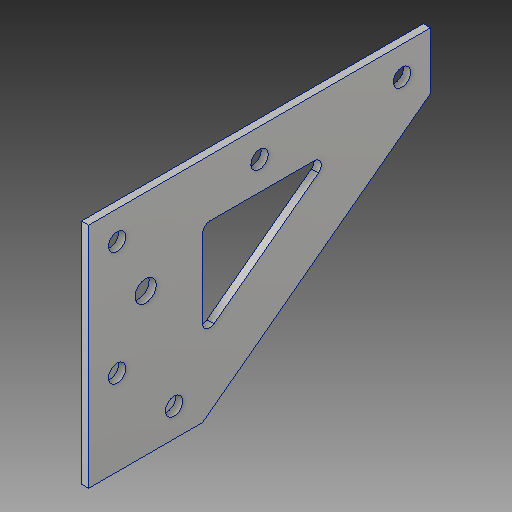
# Autodesk Inventor part: 15102898-16-P-0205
Saved by Autodesk Inventor 2017 (Build 210142000, 142)
## iProperties
Created: 2016-10-02
Part Number: 15102898-16-P-0205
Material: Aluminum 6061
Document SubType Name: Modeling
Designer: gus
Density: 2.7 g/cm^3
Appearance: Aluminum - Flat
Mass: 85.8524 g
Surface Area: 224.718 cm^2
Volume: 31.7972 cm^3
Author: gus
Autodesk Inventor part; units mm, degrees
ref_plane "YZ Plane" through (0, 0, 0) normal (1, 0, 0) x (0, 1, 0)
ref_plane "XZ Plane" through (0, 0, 0) normal (0, 1, 0) x (-1, 0, 0)
ref_plane "XY Plane" through (0, 0, 0) normal (0, 0, 1) x (1, 0, 0)
sketch "Sketch1" plane through (0, 0, 0) normal (1, 0, 0) x (0, 1, 0)
  line L0 (0, 0) -> (0, -152.4)
  line L1 (0, -152.4) -> (-25.4, -152.4)
  line L2 (-25.4, -152.4) -> (-101.6, -50.8)
  line L3 (-101.6, -50.8) -> (-101.6, 0)
  line L4 (-101.6, 0) -> (0, 0)
  circle A0 centre (-63.5, -12.7) radius 3.8956
  circle A1 centre (-12.7, -12.7) radius 3.8956
  circle A2 centre (-12.7, -76.2) radius 3.8956
  circle A3 centre (-12.7, -139.7) radius 3.8956
  line L5 (-12.7, 0) -> (-12.7, -152.4) construction
  line L6 (0, -12.7) -> (-2.3722, -12.7) construction
  line L7 (-2.3722, -12.7) -> (-101.6, -12.7) construction
  circle A4 centre (-88.9, -38.1) radius 3.8956
  circle A5 centre (-38.1, -25.4) radius 4.7625
  dimension "d0" = 50.8
  dimension "d1" = 25.4
  dimension "d2" = 101.6
  dimension "d3" = 152.4
  dimension "d4" = 63.5
  dimension "d5" = 63.5
  dimension "d6" = 12.7
  dimension "d7" = 12.7
  dimension "d8" = 50.8
  dimension "d10" = 12.7
  dimension "d11" = 12.7
  dimension "d12" = 38.1
  dimension "d13" = 9.525
  dimension "d14" = 25.4
  dimension "d15" = 7.7912
  constraints: 16 end point, 7 point on line, 6 centre point, 5 perpendicular, 4 equal radius, 2 midpoint, 2 vertical
  measures "d0" distance of L2.end L3.end
  measures "d1" distance of L0.end L1.end
  measures "d2" distance of L3.end L0.start
  measures "d3" distance of L0.start L0.end
  measures "d4" distance of A2.centre A1.centre
  measures "d5" distance of A3.centre A2.centre
  measures "d6" distance between parallel lines of L0 L5
  measures "d7" distance between parallel lines of L4 L7
  measures "d8" distance of A0.centre A1.centre
  measures "d10" distance from line of L3 A4.centre
  measures "d11" horizontal distance of A4.centre L2.end
  measures "d12" distance from line of L0 A5.centre
  measures "d13" diameter of A5
  measures "d14" distance from line of L4 A5.centre
  measures "d15" diameter of A2
extrude "Extrusion1" add sketch "Sketch1" along normal blind 3.175
sketch "Sketch2" plane through (3.175, 0, 0) normal (1, 0, 0) x (0, 0, -1)
  line L0 (50.8, -63.5) -> (50.8, -28.575)
  line L1 (53.975, -25.4) -> (100.5417, -25.4)
  line L2 (102.4467, -31.115) -> (55.88, -66.04)
  line L3 (152.4, 0) -> (0, 0) projected
  line L4 (0, 0) -> (0, -101.6) projected
  line L5 (50.8, -101.6) -> (152.4, -25.4) projected
  arc A0 (50.8, -63.5) -> (55.88, -66.04) centre (53.975, -63.5) ccw
  arc A1 (53.975, -25.4) -> (50.8, -28.575) centre (53.975, -28.575) ccw
  arc A2 (102.4467, -31.115) -> (100.5417, -25.4) centre (100.5417, -28.575) ccw
  dimension "d18" = 25.4
  dimension "d19" = 25.4
  dimension "d20" = 50.8
  dimension "d21" = 3.175
  constraints: 6 end point, 6 point on circle, 6 tangent, 3 centre point, 3 parallel, 2 equal radius
  measures "d18" distance between parallel lines of L2 L5
  measures "d19" distance between parallel lines of L3 L1
  measures "d20" distance between parallel lines of L4 L0
  measures "d21" radius of A0
extrude "Extrusion2" cut sketch "Sketch2" against normal blind 3.175
body "Solid1"
